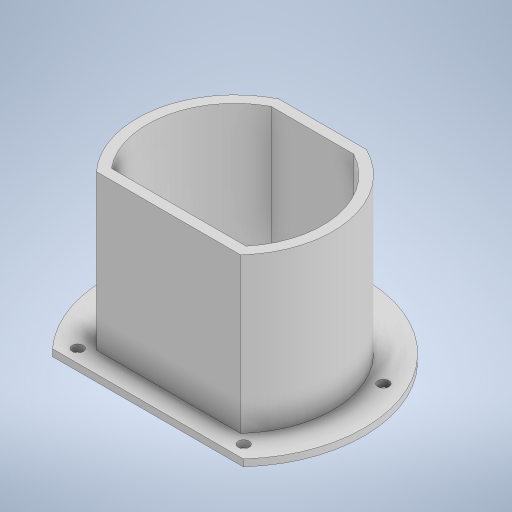
# Autodesk Inventor part: para-pocket
Saved by Autodesk Inventor 2024 (Build 280153000, 153)
## iProperties
Created: 2024-02-22
Part Number: para-pocket
Material: 一般
Document SubType Name: Modeling
Designer: mott1
Density: 1 g/cm^3
Appearance: 既定
Author: mott1
Autodesk Inventor part; units mm, degrees
ref_plane "YZ Plane" through (0, 0, 0) normal (1, 0, 0) x (0, 1, 0)
ref_plane "XZ Plane" through (0, 0, 0) normal (0, 1, 0) x (-1, 0, 0)
ref_plane "XY Plane" through (0, 0, 0) normal (0, 0, 1) x (1, 0, 0)
sketch "スケッチ1" plane through (0, 0, 0) normal (0, 1, 0) x (-1, 0, 0)
  arc A0 (-27.7473, 25.3346) -> (0, -37.5733) centre (0, 0) ccw
  line L0 (0, 0) -> (0, 25.3346)
  line L1 (0, 25.3346) -> (-27.7473, 25.3346)
  line L2 (0, 25.3346) -> (0, -37.5733)
  line L3 (0, 0) -> (-29.21, 0)
  line L4 (-29.21, 0) -> (-29.21, -13.97)
  circle A1 centre (-29.21, -13.97) radius 1.6
  line L5 (0, 0) -> (-24.13, 0)
  line L6 (-24.13, 0) -> (-24.13, 21.59)
  circle A2 centre (-24.13, 21.59) radius 1.6
  dimension "d2" = 37.5733
  dimension "d3" = 29.21
  dimension "d4" = 13.97
  dimension "d5" = 3.2
  dimension "d6" = 24.13
  dimension "d7" = 21.59
  dimension "d8" = 3.2
  constraints: 14 end point, 3 centre point, 3 coincident, 2 perpendicular, 2 point on circle, 1 point on line, 1 vertical
  measures "d2" radius of A0
  measures "d3" distance of L0.start L3.end
  measures "d4" distance of L3.end L4.end
  measures "d5" diameter of A1
  measures "d6" distance of L0.start L5.end
  measures "d7" distance of L5.end L6.end
  measures "d8" diameter of A2
extrude "押し出し1" add sketch "スケッチ1" along normal blind 2
sketch "スケッチ2" plane through (0, 2, 0) normal (0, 1, 0) x (1, 0, 0)
  arc A0 (20.9386, -19.3346) -> (12.7279, 25.5) centre (0, 0) ccw
  line L0 (0, -19.3346) -> (20.9386, -19.3346)
  line L1 (0, -25.3346) -> (27.7473, -25.3346) projected
  arc A1 (19.5814, -16.3346) -> (12, 22.5) centre (0, 0) ccw
  line L2 (0, -16.3346) -> (19.5814, -16.3346)
  line L3 (0, 37.5733) -> (0, -25.3346) projected
  line L4 (0, 28.5) -> (0, -25.3346)
  line L5 (0, 0) -> (25.5, 0)
  line L6 (0, 0) -> (0, 16.335)
  line L7 (0, 37.5733) -> (0, 25.5)
  line L8 (0, 25.5) -> (12.7279, 25.5)
  line L9 (0, 22.5) -> (12, 22.5)
  dimension "d12" = 6
  dimension "d13" = 3
  dimension "d14" = 3
  dimension "d15" = 25.5
  dimension "d20" = 3
  dimension "d21" = 28.5
  dimension "d23" = 12.0733
  dimension "d26" = 22.5
  dimension "d27" = 16.3346
  constraints: 16 end point, 5 point on circle, 4 point on line, 3 horizontal, 2 centre point, 2 coincident, 2 collinear, 1 parallel, 1 perpendicular, 1 tangent
  measures "d12" distance between parallel lines of L1 L0
  measures "d13" radial gap between concentric circles of A0 A1
  measures "d14" distance between parallel lines of L0 L2
  measures "d15" radius of A1
  measures "d20" distance between parallel lines of L8 L9
  measures "d21" radius of A0
  measures "d23" distance of L3.start L7.end
  measures "d26" distance from line of L9 point (0, 0)
  measures "d27" distance between parallel lines of L5 L2
extrude "押し出し2" add sketch "スケッチ2" along normal blind 45 contours L0 L3 L2 A1 L9 L8 A0
mirror "ミラー1" about plane through (0, 0, -37.5733) normal (-1, 0, 0) of "押し出し2", "押し出し1"
